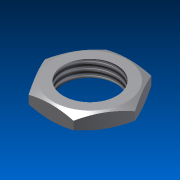
# Autodesk Inventor part: Part81
Saved by Autodesk Inventor 2014 (Build 180170000, 170)
## iProperties
Created: 2011-11-08
Part Number: Part81
Document SubType Name: Modeling
Designer: sdarley
Density: 1 g/cm^3
Material: Generic
Appearance: Default
Author: sdarley
Autodesk Inventor part; units mm, degrees
ref_plane "YZ Plane" through (0, 0, 0) normal (1, 0, 0) x (0, 1, 0)
ref_plane "XZ Plane" through (0, 0, 0) normal (0, 1, 0) x (-1, 0, 0)
ref_plane "XY Plane" through (0, 0, 0) normal (0, 0, 1) x (1, 0, 0)
sketch "Sketch1" plane through (0, 0, 0) normal (0, 0, 1) x (1, 0, 0)
  circle A0 centre (0, 0) radius 3.25
  line L0 (-2.75, 4.7631) -> (2.75, 4.7631)
  line L1 (2.75, 4.7631) -> (5.5, 0)
  line L2 (5.5, 0) -> (2.75, -4.7631)
  line L3 (2.75, -4.7631) -> (-2.75, -4.7631)
  line L4 (-2.75, -4.7631) -> (-5.5, 0)
  line L5 (-5.5, 0) -> (-2.75, 4.7631)
  point P0 (0, 4.7631)
  dimension "d0" = 6.5
  dimension "d1" = 120
  dimension "d2" = 120
  dimension "d3" = 120
  dimension "d4" = 5.5
  dimension "d7" = 5.5
  dimension "d12" = 5.5
  dimension "d14" = 5.5
  constraints: 12 end point, 2 parallel, 1 centre point, 1 coincident, 1 horizontal, 1 midpoint, 1 vertical alignment
  measures "d0" diameter of A0
  measures "d1" angle of L0 L1
  measures "d2" angle of L1 L2
  measures "d3" angle of L3 L4
  measures "d4" distance of L0.start L0.end
  measures "d7" distance of L4.end L0.start
  measures "d12" distance of L0.end L1.end
  measures "d14" distance of L1.end L2.end
extrude "Extrusion1" add sketch "Sketch1" along normal blind 2
thread "Thread1" size "M7x0.75" class "6H" standard "ISO Metric profile" full length
sketch "Sketch2" plane through (0, 0, 0) normal (0, 1, 0) x (-1, 0, 0)
  line L0 (5.5, 2) -> (2.75, 2) projected
  line L1 (2.75, 0) -> (2.75, 2) projected
  line L2 (5.5, 0) -> (2.75, 0) projected
  line L3 (5.5, 0) -> (5.5, 2) projected
  line L4 (5.5, 1.5) -> (5.5, 2)
  line L5 (5.5, 0) -> (5.5, 0.5)
  line L6 (5.5, 1.5) -> (4.5, 2)
  line L7 (4.5, 0) -> (5.5, 0.5)
  line L8 (4.5, 0) -> (5.5, 0)
  line L9 (5.5, 2) -> (4.5, 2)
  line L10 (0, -0.4) -> (0, 2.4) projected
  point P0 (0, 0)
  dimension "d15" = 0.5
  dimension "d16" = 0.5
  dimension "d17" = 1
  dimension "d18" = 1
  constraints: 12 end point, 4 point on line, 3 collinear
  measures "d15" distance from line of L0 L4.start
  measures "d16" distance from line of L5.end L2
  measures "d17" distance from line of L3 L6.end
  measures "d18" distance from line of L3 L7.start
revolve "Revolution1" cut sketch "Sketch2" angle 360 about axis through (0, 0, -10) along (0, 0, 1) contours L3 L6 L0 | L3 L2 L7
equation "\"d7\" = d4"
equation "\"d12\" = d4"
equation "\"d14\" = d4"
equation "\"d16\" = d15"
equation "\"d18\" = d17"
body "Solid1"
